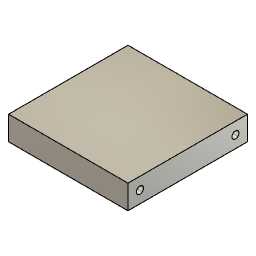
Plateau chauffant v5 (Autodesk Fusion 360 design; units mm, degrees)
Autodesk Fusion 360 part; units mm, degrees
note: some values were not read from the file. Set by a fixed rule: which sketch regions a step uses.
sketch "Esquisse1" plane through (0, 0, 0) normal (0, 1, 0) x (1, 0, 0)
  line L0 (0, 0) -> (100, 0)
  line L1 (100, 0) -> (100, 100)
  line L2 (100, 100) -> (0, 100)
  line L3 (0, 100) -> (0, 0)
  dimension "d1" = 100
  dimension "d2" = 100
  constraint horizontal L0
  constraint vertical L1
  constraint horizontal L2
  constraint vertical L3
  constraint coincident L0.start L3.end
  measures "d1" distance of L0.start L2.end
  measures "d2" distance of L0.start L0.end
extrude "Extrusion1" add sketch "Esquisse1" along normal blind 20
sketch "Esquisse2" plane through (100, 0, 0) normal (1, 0, 0) x (0, 0, -1)
  line L0 (0, 0) -> (100, 0)
  line L1 (100, 0) -> (100, 20)
  line L2 (100, 20) -> (0, 20)
  line L3 (0, 20) -> (0, 0)
  line L4 (0, 10) -> (37, 10)
  circle A0 centre (10, 10) radius 3
  line L5 (50, 20) -> (50, 0)
  circle A1 centre (90, 10) radius 3
  dimension "d5" = 6
  dimension "d6" = 10
  constraint midpoint L3 L4.start
  constraint perpendicular L3 L4
  constraint coincident L4 A0.centre
  constraint midpoint L2 L5.start
  constraint midpoint L0 L5.end
  constraint symmetric A0 L5 A1
  measures "d5" diameter of A0
  measures "d6" distance of L4.start A0.centre
extrude "Extrusion2" cut sketch "Esquisse2" against normal blind 10 contours L4 A0 | L4 A0 | A1
sketch "Esquisse3" plane through (0, 0, 0) normal (-1, 0, 0) x (0, 0, 1)
  line L0 (-100, 0) -> (0, 0)
  line L1 (0, 0) -> (0, 20)
  line L2 (0, 20) -> (-100, 20)
  line L3 (-100, 20) -> (-100, 0)
  line L4 (-100, 10) -> (-70, 10)
  line L5 (-50, 20) -> (-50, 0)
  circle A0 centre (-90, 10) radius 3
  circle A1 centre (-10, 10) radius 3
  dimension "d9" = 6
  dimension "d10" = 10
  constraint midpoint L3 L4.start
  constraint perpendicular L3 L4
  constraint midpoint L2 L5.start
  constraint midpoint L0 L5.end
  constraint coincident L4 A0.centre
  constraint symmetric L5 A0 A1
  measures "d9" diameter of A0
  measures "d10" distance of L4.start A0.centre
extrude "Extrusion3" cut sketch "Esquisse3" against normal blind 10 contours L4 A0 | L4 A0 | A1
sketch "Esquisse4" plane through (0, 0, 0) normal (0, -1, 0) x (1, 0, 0)
  line L0 (0, 0) -> (0, -100)
  line L1 (0, -100) -> (100, -100)
  line L2 (100, -100) -> (100, 0)
  line L3 (100, 0) -> (0, 0)
  line L4 (0, -5) -> (20, -5)
  line L5 (20, -5) -> (20, 0)
  line L6 (80, 0) -> (80, -5)
  line L7 (80, -5) -> (100, -5)
  line L8 (0, -95) -> (20, -95)
  line L9 (20, -95) -> (20, -100)
  line L10 (80, -100) -> (80, -95)
  line L11 (80, -95) -> (100, -95)
  line L12 (20, -5) -> (80, -5)
  line L13 (80, -95) -> (20, -95)
  line L14 (20, -95) -> (20, -5)
  line L15 (80, -5) -> (80, -95)
  line L16 (20, -90) -> (25, -90)
  line L17 (25, -90) -> (25, -95)
  line L18 (80, -90) -> (75, -90)
  line L19 (75, -90) -> (75, -95)
  circle A0 centre (25, -90) radius 1.5
  circle A1 centre (75, -90) radius 1.5
  line L20 (20, -10) -> (25, -10)
  line L21 (25, -10) -> (25, -5)
  line L22 (75, -5) -> (75, -10)
  line L23 (75, -10) -> (80, -10)
  circle A2 centre (25, -10) radius 1.5
  circle A3 centre (75, -10) radius 1.5
  line L24 (35.75, -100) -> (35.75, -75)
  line L25 (35.75, -75) -> (0, -75)
  line L26 (35.75, 0) -> (35.75, -25)
  line L27 (35.75, -25) -> (0, -25)
  line L28 (64.25, 0) -> (64.25, -25)
  line L29 (64.25, -25) -> (100, -25)
  line L30 (100, -75) -> (64.25, -75)
  line L31 (64.25, -75) -> (64.25, -100)
  line L32 (64.25, -75) -> (35.75, -75)
  line L33 (35.75, -75) -> (35.75, -25)
  line L34 (35.75, -25) -> (64.25, -25)
  line L35 (64.25, -25) -> (64.25, -75)
  line L36 (61.5, -75) -> (61.5, -72.25)
  line L37 (61.5, -72.25) -> (64.25, -72.25)
  line L38 (38.5, -75) -> (38.5, -72.25)
  line L39 (38.5, -72.25) -> (35.75, -72.25)
  line L40 (38.5, -25) -> (38.5, -27.75)
  line L41 (38.5, -27.75) -> (35.75, -27.75)
  line L42 (61.5, -25) -> (61.5, -27.75)
  line L43 (61.5, -27.75) -> (64.25, -27.75)
  circle A4 centre (38.5, -72.25) radius 1.5
  circle A5 centre (61.5, -72.25) radius 1.5
  circle A6 centre (38.5, -27.75) radius 1.5
  circle A7 centre (61.5, -27.75) radius 1.5
  dimension "d13" = 5
  dimension "d14" = 20
  dimension "d15" = 5
  dimension "d16" = 20
  dimension "d17" = 20
  dimension "d18" = 20
  dimension "d19" = 5
  dimension "d20" = 5
  dimension "d21" = 5
  dimension "d22" = 5
  dimension "d23" = 5
  dimension "d24" = 5
  dimension "d25" = 3
  dimension "d26" = 3
  dimension "d27" = 5
  dimension "d28" = 5
  dimension "d29" = 5
  dimension "d30" = 5
  dimension "d31" = 3
  dimension "d32" = 3
  dimension "d35" = 25
  dimension "d36" = 25
  dimension "d37" = 35.75
  dimension "d38" = 35.75
  dimension "d39" = 25
  dimension "d40" = 25
  dimension "d41" = 35.75
  dimension "d42" = 35.75
  dimension "d43" = 2.75
  dimension "d44" = 2.75
  dimension "d45" = 2.75
  dimension "d46" = 2.75
  dimension "d47" = 2.75
  dimension "d48" = 2.75
  dimension "d49" = 2.75
  dimension "d50" = 2.75
  dimension "d51" = 3
  dimension "d52" = 3
  dimension "d53" = 3
  dimension "d54" = 3
  constraint coincident L0 L4.start
  constraint perpendicular L0 L4
  constraint coincident L3 L5.end
  constraint perpendicular L3 L5
  constraint coincident L3 L6.start
  constraint perpendicular L3 L6
  constraint coincident L2 L7.end
  constraint perpendicular L2 L7
  constraint coincident L0 L8.start
  constraint perpendicular L0 L8
  constraint coincident L1 L9.end
  constraint perpendicular L1 L9
  constraint coincident L1 L10.start
  constraint perpendicular L1 L10
  constraint coincident L2 L11.end
  constraint perpendicular L2 L11
  constraint coincident L14 L16.start
  constraint perpendicular L14 L16
  constraint coincident L13 L17.end
  constraint perpendicular L13 L17
  constraint coincident L15 L18.start
  constraint perpendicular L15 L18
  constraint coincident L13 L19.end
  constraint perpendicular L13 L19
  constraint coincident L16.end L17.start
  constraint coincident L18.end L19.start
  constraint coincident L14 L20.start
  constraint perpendicular L14 L20
  constraint coincident L12 L21.end
  constraint perpendicular L12 L21
  constraint coincident L12 L22.start
  constraint perpendicular L12 L22
  constraint coincident L15 L23.end
  constraint perpendicular L15 L23
  constraint coincident L20.end L21.start
  constraint coincident L22.end L23.start
  constraint coincident L1 L24.start
  constraint perpendicular L1 L24
  constraint coincident L0 L25.end
  constraint perpendicular L0 L25
  constraint coincident L3 L26.start
  constraint perpendicular L3 L26
  constraint coincident L0 L27.end
  constraint perpendicular L0 L27
  constraint coincident L3 L28.start
  constraint perpendicular L12 L28
  constraint coincident L2 L29.end
  constraint perpendicular L2 L29
  constraint coincident L2 L30.start
  constraint perpendicular L15 L30
  constraint coincident L1 L31.end
  constraint perpendicular L1 L31
  constraint coincident L32 L36.start
  constraint perpendicular L32 L36
  constraint coincident L35 L37.end
  constraint perpendicular L35 L37
  constraint coincident L32 L38.start
  constraint perpendicular L32 L38
  constraint coincident L33 L39.end
  constraint perpendicular L33 L39
  constraint coincident L34 L40.start
  constraint perpendicular L34 L40
  constraint coincident L33 L41.end
  constraint perpendicular L33 L41
  constraint coincident L34 L42.start
  constraint perpendicular L34 L42
  constraint coincident L35 L43.end
  constraint perpendicular L35 L43
  constraint coincident L38.end L39.start
  constraint coincident L36.end L37.start
  constraint coincident L40.end L41.start
  constraint coincident L42.end L43.start
  measures "d13" distance of L4.end L5.end
  measures "d14" distance of L4.start L4.end
  measures "d15" distance of L6.start L6.end
  measures "d16" distance of L6.end L7.end
  measures "d17" distance of L10.end L11.end
  measures "d18" distance of L8.start L8.end
  measures "d19" distance of L8.end L9.end
  measures "d20" distance of L10.start L10.end
  measures "d21" distance of L18.start L18.end
  measures "d22" distance of L18.end L19.end
  measures "d23" distance of L16.start L16.end
  measures "d24" distance of L16.end L17.end
  measures "d25" diameter of A0
  measures "d26" diameter of A1
  measures "d27" distance of L20.end L21.end
  measures "d28" distance of L20.start L20.end
  measures "d29" distance of L22.start L22.end
  measures "d30" distance of L22.end L23.end
  measures "d31" diameter of A2
  measures "d32" diameter of A3
  measures "d35" distance of L30.end L31.end
  measures "d36" distance of L24.start L24.end
  measures "d37" distance of L30.start L30.end
  measures "d38" distance of L24.end L25.end
  measures "d39" distance of L28.start L28.end
  measures "d40" distance of L26.start L26.end
  measures "d41" distance of L28.end L29.end
  measures "d42" distance of L26.end L27.end
  measures "d43" distance of L42.end L43.end
  measures "d44" distance of L42.start L42.end
  measures "d45" distance of L40.start L40.end
  measures "d46" distance of L40.end L41.end
  measures "d47" distance of L38.end L39.end
  measures "d48" distance of L38.start L38.end
  measures "d49" distance of L36.start L36.end
  measures "d50" distance of L36.end L37.end
  measures "d51" diameter of A5
  measures "d52" diameter of A4
  measures "d53" diameter of A7
  measures "d54" diameter of A6
extrude "Extrusion4" cut sketch "Esquisse4" against normal blind 10 contours L20 L21 A2 | L20 L21 A2 | L16 L17 A0 | L16 L17 A0 | L22 L23 A3 | L22 L23 A3 | L18 L19 A1 | L18 L19 A1
extrude "Extrusion5" cut sketch "Esquisse4" against normal blind 10 contours L40 L41 A6 | L40 L41 A6 | L38 L39 A4 | L38 L39 A4 | L42 L43 A7 | L42 L43 A7 | L36 L37 A5 | L36 L37 A5
